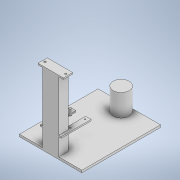
# Autodesk Inventor part: main_stand_lower_half
Saved by Autodesk Inventor 2021 (Build 250183000, 183)
## iProperties
Created: 2020-10-09
Part Number: main_stand_lower_half
Material: Generic
Document SubType Name: Modeling
Designer: bober
Density: 1 g/cm^3
Appearance: Default
Author: bober
Autodesk Inventor part; units mm, degrees
ref_plane "YZ Plane" through (0, 0, 0) normal (1, 0, 0) x (0, 1, 0)
ref_plane "XZ Plane" through (0, 0, 0) normal (0, 1, 0) x (-1, 0, 0)
ref_plane "XY Plane" through (0, 0, 0) normal (0, 0, 1) x (1, 0, 0)
sketch "Sketch1" plane through (0, 0, 0) normal (0, 1, 0) x (-1, 0, 0)
  circle A0 centre (0, 0) radius 17.5
  dimension "d0" = 35
  constraints: 1 centre point, 1 coincident
  measures "d0" diameter of A0
extrude "Extrusion1" add sketch "Sketch1" along normal blind 48
sketch "Sketch2" plane through (0, 0, 0) normal (0, -1, 0) x (1, 0, 0)
  line L0 (17.5, -17.5) -> (-17.5, -17.5)
  line L1 (-17.5, -17.5) -> (-17.5, 152.5)
  line L2 (-17.5, 152.5) -> (17.5, 152.5)
  line L3 (17.5, 152.5) -> (17.5, -17.5)
  point P0 (0, 0)
  dimension "d3" = 170
  constraints: 8 end point, 2 parallel, 1 horizontal, 1 perpendicular
  measures "d3" distance of L0.end L1.end
extrude "Extrusion2" add sketch "Sketch2" along normal blind 5
sketch "Sketch3" plane through (0, 0, 0) normal (0, 1, 0) x (1, 0, 0)
  line L0 (17.5, -152.5) -> (-17.5, -152.5) projected
  line L1 (-17.5, -152.5) -> (-17.5, 17.5) projected
  line L2 (17.5, -152.5) -> (-17.5, -152.5)
  line L3 (-17.5, -152.5) -> (-17.5, -132.5)
  line L4 (-17.5, -132.5) -> (17.5, -132.5)
  line L5 (17.5, -132.5) -> (17.5, -152.5)
  point P0 (0, 0)
  dimension "d6" = 20
  constraints: 8 end point, 2 parallel, 1 horizontal, 1 perpendicular, 1 point on line
  measures "d6" distance of L2.end L3.end
extrude "Extrusion3" add sketch "Sketch3" along normal blind 150
sketch "Sketch4" plane through (0, 48, 0) normal (0, 1, 0) x (1, 0, 0)
  line L0 (0, 0) -> (0, -110)
  circle A0 centre (0, -110) radius 2.4
  dimension "d9" = 110
  dimension "d10" = 4.8
  constraints: 2 end point, 1 centre point, 1 coincident, 1 vertical
  measures "d9" distance of L0.start L0.end
  measures "d10" diameter of A0
extrude "Extrusion4" add sketch "Sketch4" along normal blind 13
sketch "Sketch5" plane through (17.5, 0, 0) normal (1, 0, 0) x (0, 0, -1)
  line L0 (-152.5, 150) -> (-152.5, -5) projected
  line L1 (-152.5, 37.2) -> (-92.5, 37.2)
  line L2 (-92.5, 37.2) -> (-92.5, 40.2)
  line L3 (-92.5, 40.2) -> (-152.5, 40.2)
  line L4 (-152.5, 40.2) -> (-152.5, 37.2)
  point P0 (0, 0)
  dimension "d13" = 60
  dimension "d14" = 3
  constraints: 8 end point, 2 parallel, 1 horizontal, 1 perpendicular, 1 point on line
  measures "d13" distance of L3.end L2.end
  measures "d14" distance of L2.end L1.end
extrude "Extrusion5" add sketch "Sketch5" along normal blind 5
sketch "Sketch7" plane through (17.5, 40.2, 132.5) normal (0, 1, 0) x (1, 0, 0)
  line L0 (-33.3, 6.6) -> (-1.7, 6.6)
  line L1 (-1.7, 6.6) -> (-1.7, 38.4)
  line L2 (-1.7, 38.4) -> (-33.3, 38.4)
  line L3 (-33.3, 38.4) -> (-33.3, 6.6)
  circle A0 centre (-17.5, 22.5) radius 2.4 projected
  line L4 (-33.3, 6.6) -> (-1.7, 38.4) construction
  line L5 (-1.7, 6.6) -> (-33.3, 38.4) construction
  circle A1 centre (-1.7, 38.4) radius 1.5
  circle A2 centre (-1.7, 6.6) radius 1.5
  circle A3 centre (-33.3, 6.6) radius 1.5
  circle A4 centre (-33.3, 38.4) radius 1.5
  point P0 (-17.5, 132.5)
  dimension "d19" = 31.6
  dimension "d20" = 31.8
  dimension "d21" = 3
  dimension "d22" = 3
  dimension "d23" = 3
  dimension "d24" = 3
  constraints: 12 end point, 4 centre point, 3 coincident, 2 midpoint, 2 parallel, 1 horizontal, 1 perpendicular, 1 point on line
  measures "d19" distance of L2.end L1.end
  measures "d20" distance of L1.end L0.end
  measures "d21" diameter of A1
  measures "d22" diameter of A2
  measures "d23" diameter of A3
  measures "d24" diameter of A4
sketch "Sketch8" plane through (17.5, 40.2, 132.5) normal (0, 1, 0) x (1, 0, 0)
  line L0 (5, 40) -> (5, -20) projected
  line L1 (5, -20) -> (-7, -20)
  line L2 (-7, -20) -> (-7, 45)
  line L3 (-7, 45) -> (5, 45)
  line L4 (5, 45) -> (5, -20)
  point P0 (-17.5, 132.5)
  dimension "d25" = 12
  dimension "d26" = 65
  constraints: 8 end point, 2 parallel, 1 horizontal, 1 perpendicular
  measures "d25" distance of L2.end L3.end
  measures "d26" distance of L1.end L2.end
extrude "Extrusion7" add sketch "Sketch8" against normal blind 3
sketch "Sketch9" plane through (17.5, 40.2, 152.5) normal (0, 1, 0) x (1, 0, 0)
  line L0 (-40, 0) -> (-28, 0)
  line L1 (-28, 0) -> (-28, 65)
  line L2 (-28, 65) -> (-40, 65)
  line L3 (-40, 65) -> (-40, 0)
  point P0 (-17.5, 152.5)
  dimension "d29" = 12
  constraints: 8 end point, 2 parallel, 1 horizontal, 1 perpendicular
  measures "d29" distance of L2.end L1.end
extrude "Extrusion8" add sketch "Sketch9" against normal blind 3
extrude "Extrusion9" cut sketch "Sketch7" against normal blind 3 contours L3 A3 L0 | L0 A3 L3 | A2 L1 L0 | L0 L1 A2 | A4 L2 L3 | L3 L2 A4 | A1 L2 L1 | L1 L2 A1
sketch "Sketch10" plane through (0, 150, 0) normal (0, 1, 0) x (1, 0, 0)
  line L0 (27.5, -152.5) -> (-27.5, -152.5)
  line L1 (-27.5, -152.5) -> (-27.5, -132.5)
  line L2 (-27.5, -132.5) -> (27.5, -132.5)
  line L3 (27.5, -132.5) -> (27.5, -152.5)
  point P0 (0, 0)
  dimension "d34" = 55
  constraints: 8 end point, 2 parallel, 1 horizontal, 1 perpendicular
  measures "d34" distance of L1.end L2.end
extrude "Extrusion10" add sketch "Sketch10" along normal blind 3
sketch "Sketch11" plane through (0, 153, 0) normal (0, 1, 0) x (1, 0, 0)
  circle A0 centre (-22.5, -142.5) radius 2
  circle A1 centre (22.5, -142.5) radius 2
  point P0 (0, 0)
  dimension "d37" = 4
  dimension "d38" = 4
  constraints: 2 centre point
  measures "d37" diameter of A0
  measures "d38" diameter of A1
extrude "Extrusion11" cut sketch "Sketch11" against normal blind 3
sketch "Sketch12" plane through (17.5, 0, 0) normal (1, 0, 0) x (0, 0, -1)
  line L0 (17.5, 0) -> (17.5, -5) projected
  line L1 (17.5, -5) -> (-152.5, -5)
  line L2 (-152.5, -5) -> (-152.5, 0)
  line L3 (-152.5, 0) -> (17.5, 0)
  line L4 (17.5, 0) -> (17.5, -5)
  point P0 (0, 0)
  constraints: 8 end point, 2 parallel, 1 horizontal, 1 perpendicular
extrude "Extrusion12" add sketch "Sketch12" along normal blind 50 and the other way blind 85
body "Solid1"
